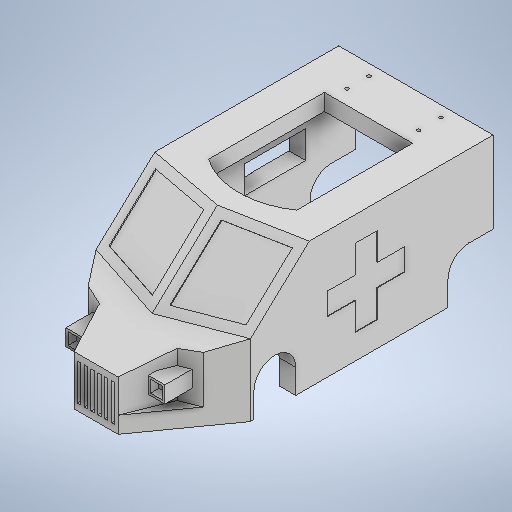
# Autodesk Inventor part: car_cover
Saved by Autodesk Inventor 2025 (Build 290162010, 162A)
## iProperties
Created: 2024-10-24
Part Number: car_cover
Material: Generic
Document SubType Name: Modeling
Designer: fist5
Density: 1 g/cm^3
Appearance: Default
Author: fist5
Autodesk Inventor part; units mm, degrees
sketch "Sketch1" plane through (0, 0, 0) normal (0, 1, 0) x (-1, 0, 0)
  line L0 (0, 0) -> (-140, 0)
  line L1 (-140, 0) -> (-140, -290)
  line L2 (-140, -290) -> (0, -290)
  line L3 (0, -290) -> (0, 0)
  line L4 (0, -70) -> (-50, 0)
  line L5 (-90, 0) -> (-140, -70)
  dimension "d0" = 290
  dimension "d1" = 140
  dimension "d2" = 70
  dimension "d3" = 50
  dimension "d4" = 50
  constraints: 12 end point, 4 point on line, 2 parallel, 1 horizontal, 1 horizontal alignment, 1 perpendicular
  measures "d0" distance between parallel lines of L2 L0
  measures "d1" distance between parallel lines of L1 L3
  measures "d2" vertical distance of L4.end L4.start
  measures "d3" distance of L0.start L4.end
  measures "d4" distance of L0.end L5.start
extrude "Extrusion1" add sketch "Sketch1" along normal blind 115 contours L4 L3 L2 L1 L5 L0
sketch "Sketch2" plane through (140, 0, -70) normal (1, 0, 0) x (0, 0, -1)
  line L0 (-70, 0) -> (-70, 115) projected
  line L1 (-70, 45) -> (0, 65)
  line L2 (0, 0) -> (0, 115) projected
  line L3 (0, 65) -> (40, 115)
  line L4 (220, 115) -> (0, 115) projected
  line L5 (-70, 0) -> (0, 0) projected
  line L6 (0, 0) -> (0, 115) projected
  line L7 (-70, 115) -> (0, 115) projected
  line L8 (-70, 0) -> (-70, 115) projected
  point P0 (0, 115)
  dimension "d7" = 20
  dimension "d8" = 45
  dimension "d9" = 40
  constraints: 4 end point, 3 point on line
  measures "d7" vertical distance of L1.start L1.end
  measures "d8" distance of L0.start L1.start
  measures "d9" horizontal distance of L3.end L1.end
extrude "Extrusion2" cut sketch "Sketch2" against normal up to next contours L0 L7 L2 L1
extrude "Extrusion3" cut sketch "Sketch2" against normal up to next contours L2 L4 L3
sketch "Sketch5" plane through (50, 45, 0) normal (0, 0.9615239, 0.2747211) x (1, 0, 0)
  line L0 (90, 72.8011) -> (-50, 72.8011) projected
  line L1 (-50, 298.0724) -> (-50, 124.9981) projected
  point P0 (-50, -12.3625)
  point P1 (20, 52.8011)
  dimension "d17" = 20
  dimension "d18" = 70
  measures "d17" distance from line of L0 point (20, 52.801)
  measures "d18" distance from line of L1 point (20, 52.801)
ref_plane "Work Plane2" through (70, 115, -110) normal (0.1294539, 0.7236066, 0.677964) x (0, -0.6837172, 0.7297471)
sketch "Sketch7" plane through (70, 115, -110) normal (0.1294539, 0.7236066, 0.677964) x (0, -0.6837172, 0.7297471)
  line L0 (0, -69.411) -> (0, 69.411) projected
  line L1 (0, 69.411) -> (-131.3545, 85.3428) projected
  line L2 (-131.3545, 85.3428) -> (-131.3545, -53.4792) projected
  line L3 (-131.3545, -53.4792) -> (0, -69.411) projected
  line L4 (63.3757, -68.2279) -> (0, -69.411) projected
  line L5 (63.3757, 70.594) -> (63.3757, -68.2279) projected
  line L6 (0, 69.411) -> (63.3757, 70.594) projected
  line L7 (0, -69.411) -> (0, 69.411) projected
  line L8 (0, 69.411) -> (63.3757, 70.594) projected
  line L9 (107.8174, 76.7345) -> (63.3757, 70.594) projected
  line L10 (107.8174, 76.7345) -> (-52.727, 96.2066) projected
  line L11 (-52.727, 96.2066) -> (-131.3545, 85.3428) projected
  line L12 (0, 69.411) -> (-131.3545, 85.3428) projected
  line L13 (128.1324, -22.955) -> (63.3757, -68.2279) projected
  line L14 (128.1324, 16.7084) -> (128.1324, -22.955) projected
  line L15 (63.3757, 70.594) -> (128.1324, 16.7084) projected
  line L16 (63.3757, 70.594) -> (63.3757, -68.2279) projected
  line L17 (63.3757, 70.594) -> (128.1324, 16.7084) projected
  line L18 (158.8997, 20.9595) -> (128.1324, 16.7084) projected
  line L19 (158.8997, 20.9595) -> (107.8174, 76.7345) projected
  line L20 (107.8174, 76.7345) -> (63.3757, 70.594) projected
  line L21 (128.1324, 16.7084) -> (128.1324, -22.955) projected
  line L22 (107.8174, -62.0875) -> (63.3757, -68.2279) projected
  line L23 (107.8174, -62.0875) -> (158.8997, -18.7039) projected
  line L24 (128.1324, 16.7084) -> (128.1324, -22.955) projected
  line L25 (158.8997, -18.7039) -> (128.1324, -22.955) projected
  line L26 (158.8997, -18.7039) -> (158.8997, 20.9595) projected
  line L27 (158.8997, 20.9595) -> (128.1324, 16.7084) projected
  line L28 (0, 0) -> (81.1658, 0)
  line L29 (81.1658, 0) -> (63.3757, 70.594)
  line L30 (0, 0) -> (63.3757, 70.594)
  point P0 (158.8997, -68.2832)
  constraints: 6 end point, 1 midpoint, 1 perpendicular
extrude "Extrusion4" cut sketch "Sketch7" along normal up to next contours L3 L2 L1 L0 | L0 L28 L5 L4 | L30 L5 L28 | L0 L6 L30 | L1 L11 L10 L9 L6
extrude "Extrusion5" add sketch "Sketch7" against normal blind 20 contours L30 L5 L28 | L5 L29 L28
ref_plane "Work Plane3" through (70, 115, -110) normal (0.1294539, -0.7236066, -0.677964) x (0, -0.6837172, 0.7297471)
sketch "Sketch9" plane through (70, 115, -110) normal (0.1294539, -0.7236066, -0.677964) x (0, -0.6837172, 0.7297471)
  line L0 (81.1658, 0) -> (63.3757, 2.3661) projected
  line L1 (-131.3545, 85.3428) -> (0, 69.411) projected
  line L2 (81.1658, 0) -> (0, 0)
  line L3 (0, 0) -> (0, 69.411)
  line L4 (0, 69.411) -> (81.1658, 69.411)
  line L5 (81.1658, 69.411) -> (81.1658, 0)
  line L6 (0, 0) -> (-9.7539, -68.2279) projected
  line L7 (0, 0) -> (-9.7539, -68.2279) projected
  line L8 (-9.7539, -68.2279) -> (-131.3545, -53.4792) projected
  line L9 (-131.3545, -53.4792) -> (-131.3545, 85.3428) projected
  line L10 (-131.3545, 85.3428) -> (0, 69.411) projected
  line L11 (0, 69.411) -> (0, 0) projected
  line L12 (0, 0) -> (81.1658, 0) projected
  line L13 (93.1192, -47.4335) -> (81.1658, 0) projected
  line L14 (148.2908, -20.1697) -> (93.1192, -47.4335) projected
  line L15 (153.1835, 20.1697) -> (148.2908, -20.1697) projected
  line L16 (63.3757, 70.594) -> (153.1835, 20.1697) projected
  line L17 (81.1658, 0) -> (63.3757, 70.594) projected
  line L18 (0, 0) -> (-9.7539, 70.594) projected
  line L19 (63.3757, 70.594) -> (0, 0) projected
  line L20 (-9.7539, 70.594) -> (63.3757, 70.594) projected
  line L21 (0, 0) -> (81.1658, 0) projected
  line L22 (0, 0) -> (-9.7539, 70.594) projected
  line L23 (63.3757, 70.594) -> (0, 0) projected
  line L24 (0, 0) -> (81.1658, 0) projected
  line L25 (0, 0) -> (-9.7539, 70.594) projected
  line L26 (63.3757, 70.594) -> (0, 0) projected
  line L27 (93.1192, -47.4335) -> (81.1658, 0) projected
  line L28 (148.2908, -20.1697) -> (93.1192, -47.4335) projected
  line L29 (153.1835, 20.1697) -> (148.2908, -20.1697) projected
  line L30 (63.3757, 70.594) -> (153.1835, 20.1697) projected
  line L31 (81.1658, 0) -> (63.3757, 70.594) projected
  line L32 (-9.7539, 70.594) -> (63.3757, 70.594) projected
  line L33 (93.1192, -47.4335) -> (81.1658, 0) projected
  line L34 (148.2908, -20.1697) -> (93.1192, -47.4335) projected
  line L35 (153.1835, 20.1697) -> (148.2908, -20.1697) projected
  line L36 (63.3757, 70.594) -> (153.1835, 20.1697) projected
  line L37 (81.1658, 0) -> (63.3757, 70.594) projected
  line L38 (-9.7539, 70.594) -> (63.3757, 70.594) projected
  point P0 (158.8997, 70.5388)
  point P1 (62.3137, 69.411)
  point P2 (63.6739, 69.411)
  point P3 (65.4828, 69.411)
  constraints: 8 end point, 2 parallel, 1 horizontal, 1 perpendicular, 1 point on line
extrude "Extrusion7" cut sketch "Sketch9" against normal blind 20 contours L20 L19 L4 L1 | L1 L3 L18 | L4 L19 L3
extrude "Extrusion8" add sketch "Sketch9" along normal blind 20 contours L19 L4 L17 L2 | L16 L4 L17 | L17 L4 L19 | L17 L4 L16 L5 | L5 L16 L15 L14 L13
sketch "Sketch10" plane through (140, 0, -290) normal (0, 0, -1) x (-1, 0, 0)
  line L0 (140, 0) -> (0, 0)
  line L1 (0, 0) -> (0, -20)
  line L2 (0, -20) -> (140, -20)
  line L3 (140, -20) -> (140, 0)
  dimension "d31" = 20
  constraints: 8 end point, 2 parallel, 1 horizontal, 1 perpendicular
  measures "d31" distance between parallel lines of L0 L2
extrude "Extrusion9" cut sketch "Sketch10" against normal up to next
ref_plane "Work Plane5" through (0, 15, 0) normal (0, -1, 0) x (1, 0, 0)
sketch "Sketch11" plane through (0, 15, 0) normal (0, -1, 0) x (1, 0, 0)
  line L0 (50, 0) -> (0, -70) projected
  line L1 (0, -70) -> (25, -63.132)
  line L2 (70, -50.7695) -> (0, -70) projected
  line L3 (25, -63.132) -> (50, 0)
  line L4 (90, 0) -> (140, -70) projected
  line L5 (90, 0) -> (140, -70)
  line L6 (140, -70) -> (70, -50.7695)
  line L7 (50, 0) -> (90, 0) projected
  line L8 (90, 0) -> (115, -63.132)
  line L9 (34.8321, -38.3031) -> (17.8321, -45.035)
  line L10 (105.1679, -38.3031) -> (122.1679, -45.035)
  line L11 (34.8321, -38.3031) -> (50, 0)
  line L12 (105.1679, -38.3031) -> (90, 0)
  line L13 (122.1679, -45.035) -> (90, 0)
  line L14 (17.8321, -45.035) -> (50, 0)
  point P0 (0, 0)
  dimension "d36" = 25
  dimension "d37" = 25
  dimension "d40" = 17
  dimension "d41" = 17
  constraints: 22 end point, 6 point on line, 4 collinear, 1 horizontal alignment, 1 perpendicular
  measures "d36" horizontal distance of L1.end L0.start
  measures "d37" horizontal distance of L8.end L4.start
  measures "d40" horizontal distance of L10.start L10.end
  measures "d41" horizontal distance of L9.start L9.end
extrude "Extrusion10" cut sketch "Sketch11" against normal up to next contours L3 L9 L0 | L4 L10 L8
ref_plane "Work Plane6" through (0, 35, 0) normal (0, -1, 0) x (1, 0, 0)
sketch "Sketch12" plane through (0, 35, 0) normal (0, -1, 0) x (1, 0, 0)
  line L0 (114.8999, -25) -> (99.8999, -25)
  line L1 (99.8999, -25) -> (99.8999, -50)
  line L2 (99.8999, -50) -> (114.8999, -50)
  line L3 (114.8999, -50) -> (114.8999, -25)
  line L4 (90, 0) -> (105.1679, -38.3031) projected
  line L5 (34.8321, -38.3031) -> (50, 0) projected
  line L6 (40.1001, -25) -> (25.1001, -25)
  line L7 (25.1001, -25) -> (25.1001, -50)
  line L8 (25.1001, -50) -> (40.1001, -50)
  line L9 (40.1001, -50) -> (40.1001, -25)
  point P0 (0, 0)
  point P1 (114.8999, -37.5)
  point P2 (99.8999, -37.5)
  point P3 (107.3999, -25)
  point P4 (107.3999, -50)
  point P5 (32.6001, -25)
  dimension "d43" = 15
  dimension "d44" = 25
  dimension "d45" = 25
  dimension "d46" = 15
  dimension "d47" = 25
  dimension "d48" = 25
  constraints: 16 end point, 5 midpoint, 4 parallel, 2 horizontal, 2 perpendicular, 2 point on line
  measures "d43" distance of point (114.9, -37.5) point (99.9, -37.5)
  measures "d44" distance of point (107.4, -25) point (107.4, -50)
  measures "d45" distance from line of L4.start L0
  measures "d46" distance between parallel lines of L7 L9
  measures "d47" vertical distance of point (0, 0) point (32.6, -25)
  measures "d48" distance between parallel lines of L6 L8
extrude "Extrusion11" add sketch "Sketch12" along normal blind 7.5 and the other way blind 7.5
sketch "Sketch13" plane through (25.1001, 27.5, -25) normal (0, 0, 1) x (1, 0, 0)
  line L0 (0, 15) -> (15, 15) projected
  line L1 (15, 15) -> (15, 0) projected
  line L2 (15, 0) -> (0, 0) projected
  line L3 (0, 0) -> (0, 15) projected
  line L4 (15, 15) -> (15, 24.6429) projected
  line L5 (15, 24.6429) -> (74.7998, 24.6429) projected
  line L6 (74.7998, 24.6429) -> (74.7998, 15) projected
  line L7 (74.7998, 0) -> (74.7998, 15) projected
  line L8 (89.7998, 0) -> (74.7998, 0) projected
  line L9 (89.7998, 15) -> (89.7998, 0) projected
  line L10 (74.7998, 15) -> (89.7998, 15) projected
  line L11 (15, -12.5) -> (15, 0) projected
  line L12 (7.0428, -12.5) -> (15, -12.5) projected
  line L13 (7.0428, -27.5) -> (7.0428, -12.5) projected
  line L14 (82.757, -27.5) -> (7.0428, -27.5) projected
  line L15 (82.757, -12.5) -> (82.757, -27.5) projected
  line L16 (74.7998, -12.5) -> (82.757, -12.5) projected
  line L17 (74.7998, 0) -> (74.7998, -12.5) projected
  line L18 (2, 15) -> (2, 0)
  line L19 (13, 15) -> (13, 0)
  line L20 (0, 13) -> (15, 13)
  line L21 (0, 2) -> (15, 2)
  line L22 (74.7998, 13) -> (89.7998, 13)
  line L23 (74.7998, 2) -> (89.7998, 2)
  line L24 (76.7998, 15) -> (76.7998, 0)
  line L25 (89.7998, 0) -> (80.0678, 0) projected
  line L26 (87.7998, 15) -> (87.7998, 0)
  line L27 (2, 13) -> (13, 13)
  line L28 (13, 13) -> (13, 2)
  line L29 (13, 2) -> (2, 2)
  line L30 (2, 2) -> (2, 13)
  line L31 (76.7998, 13) -> (87.7998, 13)
  line L32 (87.7998, 13) -> (87.7998, 2)
  line L33 (87.7998, 2) -> (76.7998, 2)
  line L34 (76.7998, 2) -> (76.7998, 13)
  line L35 (0, 15) -> (15, 15) projected
  line L36 (0, 15) -> (15, 15)
  line L37 (15, 15) -> (15, 0)
  line L38 (15, 0) -> (0, 0)
  line L39 (0, 0) -> (0, 15)
  line L40 (74.7998, 15) -> (80.0678, 15) projected
  line L41 (74.7998, 15) -> (89.7998, 15)
  line L42 (89.7998, 15) -> (89.7998, 0)
  line L43 (89.7998, 0) -> (74.7998, 0)
  line L44 (74.7998, 0) -> (74.7998, 15)
  point P0 (-25.1001, -27.5)
  point P1 (7.5, 0)
  point P2 (7.5, 2)
  point P3 (87.7998, 13)
  point P4 (13, 13)
  point P5 (2, 2)
  dimension "d53" = 2
  dimension "d54" = 11
  dimension "d55" = 2
  dimension "d56" = 11
  dimension "d57" = 2
  dimension "d58" = 11
  dimension "d59" = 2
  dimension "d60" = 2
  constraints: 48 end point, 24 point on line, 10 perpendicular, 8 parallel, 5 horizontal, 2 midpoint, 1 vertical
  measures "d53" distance of point (7.5, 0) point (7.5, 2)
  measures "d54" distance between parallel lines of L21 L20
  measures "d55" distance between parallel lines of L3 L18
  measures "d56" distance between parallel lines of L18 L19
  measures "d57" distance between parallel lines of L9 L26
  measures "d58" distance between parallel lines of L26 L24
  measures "d59" distance between parallel lines of L10 L22
  measures "d60" distance between parallel lines of L8 L23
extrude "Extrusion12" add sketch "Sketch13" along normal blind 7.5 contours L0 L18 L20 L3 | L0 L19 L20 L18 | L20 L18 L21 L3 | L0 L1 L20 L19 | L21 L18 L2 L3 | L20 L1 L21 L19 | L21 L19 L2 L18 | L21 L1 L2 L19 | L10 L24 L22 L7 | L22 L24 L23 L7 | L10 L26 L22 L24 | L23 L24 L8 L7 | L23 L26 L8 L24 | L26 L10 L9 L22 | L22 L9 L23 L26 | L23 L9 L8 L26
sketch "Sketch14" plane through (50, 0, 0) normal (0, 0, 1) x (1, 0, 0)
  line L0 (3.0769, 39) -> (6.1538, 39)
  line L1 (6.1538, 39) -> (6.1538, 6)
  line L2 (6.1538, 6) -> (3.0769, 6)
  line L3 (3.0769, 6) -> (3.0769, 39)
  line L4 (9.2308, 39) -> (12.3077, 39)
  line L5 (12.3077, 39) -> (12.3077, 6)
  line L6 (12.3077, 6) -> (9.2308, 6)
  line L7 (9.2308, 6) -> (9.2308, 39)
  line L8 (15.3846, 39) -> (18.4615, 39)
  line L9 (18.4615, 39) -> (18.4615, 6)
  line L10 (18.4615, 6) -> (15.3846, 6)
  line L11 (15.3846, 6) -> (15.3846, 39)
  line L12 (21.5385, 39) -> (24.6154, 39)
  line L13 (24.6154, 39) -> (24.6154, 6)
  line L14 (24.6154, 6) -> (21.5385, 6)
  line L15 (21.5385, 6) -> (21.5385, 39)
  line L16 (27.6923, 39) -> (30.7692, 39)
  line L17 (30.7692, 39) -> (30.7692, 6)
  line L18 (30.7692, 6) -> (27.6923, 6)
  line L19 (27.6923, 6) -> (27.6923, 39)
  line L20 (33.8462, 39) -> (36.9231, 39)
  line L21 (36.9231, 39) -> (36.9231, 6)
  line L22 (36.9231, 6) -> (33.8462, 6)
  line L23 (33.8462, 6) -> (33.8462, 39)
  line L24 (0, 15) -> (0, 45) projected
  line L25 (40, 45) -> (0, 45) projected
  line L26 (0, 0) -> (40, 0) projected
  point P0 (-50, 0)
  point P1 (16.9231, 39)
  point P2 (35.3846, 6)
  dimension "d63" = 3.0769
  dimension "d64" = 3.0769
  dimension "d65" = 3.0769
  dimension "d66" = 3.0769
  dimension "d67" = 3.0769
  dimension "d68" = 3.0769
  dimension "d69" = 3.0769
  dimension "d70" = 3.0769
  dimension "d71" = 3.0769
  dimension "d72" = 3.0769
  dimension "d73" = 3.0769
  dimension "d74" = 3.0769
  dimension "d75" = 6
  dimension "d76" = 6
  constraints: 48 end point, 12 parallel, 9 point on line, 6 horizontal, 6 perpendicular, 2 midpoint, 1 horizontal alignment
  measures "d63" distance between parallel lines of L24 L3
  measures "d64" distance between parallel lines of L7 L1
  measures "d65" distance between parallel lines of L11 L5
  measures "d66" distance between parallel lines of L3 L1
  measures "d67" distance between parallel lines of L11 L9
  measures "d68" distance between parallel lines of L9 L15
  measures "d69" distance between parallel lines of L7 L5
  measures "d70" distance between parallel lines of L13 L15
  measures "d71" distance between parallel lines of L13 L19
  measures "d72" distance between parallel lines of L19 L17
  measures "d73" distance between parallel lines of L17 L23
  measures "d74" distance between parallel lines of L23 L21
  measures "d75" distance from line of point (16.923, 39) L25
  measures "d76" distance from line of L26 point (35.385, 6)
extrude "Extrusion13" cut sketch "Sketch14" against normal blind 7.5
sketch "Sketch15" plane through (70, 115, -110) normal (0.1294539, 0.7236066, 0.677964) x (0.9915854, -0.0944686, -0.0885098)
  line L0 (8, -6.9706) -> (62.594, 0.5726)
  line L1 (62.594, 0.5726) -> (62.594, -57.1417)
  line L2 (62.594, -57.1417) -> (8, -70.8996)
  line L3 (8, -70.8996) -> (8, -6.9706)
  line L4 (0, 0) -> (0, -81.1658) projected
  line L5 (0, 0) -> (70.594, 9.7539) projected
  line L6 (70.594, 9.7539) -> (70.594, -63.3757) projected
  line L7 (70.594, -63.3757) -> (0, -81.1658) projected
  point P0 (-68.2832, -158.8997)
  dimension "d79" = 8
  dimension "d80" = 8
  dimension "d81" = 8
  dimension "d82" = 8
  constraints: 8 end point, 4 parallel
  measures "d79" distance between parallel lines of L5 L0
  measures "d80" distance between parallel lines of L6 L1
  measures "d81" distance between parallel lines of L7 L2
  measures "d82" distance between parallel lines of L4 L3
extrude "Extrusion14" cut sketch "Sketch15" against normal blind 1 contours L0 L1 L2 L3
sketch "Sketch16" plane through (70, 115, -110) normal (-0.1294539, 0.7236066, 0.677964) x (0.9915854, 0.0944686, 0.0885098)
  line L0 (-8, -70.8996) -> (-62.594, -57.1417)
  line L1 (-62.594, -57.1417) -> (-62.594, 0.5726)
  line L2 (-62.594, 0.5726) -> (-8, -6.9706)
  line L3 (-8, -6.9706) -> (-8, -70.8996)
  line L4 (-70.594, 9.7539) -> (0, 0) projected
  line L5 (0, 0) -> (0, -81.1658) projected
  line L6 (0, -81.1658) -> (-70.594, -63.3757) projected
  line L7 (-70.594, -63.3757) -> (-70.594, 9.7539) projected
  point P0 (-70.5388, -158.8997)
  point P1 (0, -40.5829)
  dimension "d85" = 8
  dimension "d86" = 8
  dimension "d87" = 8
  dimension "d88" = 8
  constraints: 8 end point, 5 parallel, 1 midpoint, 1 vertical
  measures "d85" distance between parallel lines of L4 L2
  measures "d86" distance between parallel lines of L7 L1
  measures "d87" distance between parallel lines of L6 L0
  measures "d88" distance from line of point (0, -40.583) L3
extrude "Extrusion15" cut sketch "Sketch16" against normal blind 1 contours L0 L1 L2 L3
sketch "Sketch17" plane through (0, 0, 0) normal (0, -1, 0) x (1, 0, 0)
  line L0 (90, 0) -> (140, -70) projected
  line L1 (140, -70) -> (140, -290) projected
  line L2 (140, -290) -> (0, -290) projected
  line L3 (0, -290) -> (0, -70) projected
  line L4 (0, -70) -> (50, 0) projected
  line L5 (50, 0) -> (90, 0) projected
  line L6 (0, -123.3662) -> (70, -110) projected
  line L7 (70, -110) -> (140, -123.3662) projected
  line L8 (140, -123.3662) -> (140, -290) projected
  line L9 (140, -290) -> (0, -290) projected
  line L10 (0, -290) -> (0, -123.3662) projected
  line L11 (125, -290) -> (15, -290)
  line L12 (15, -290) -> (15, -120.502)
  line L13 (15, -120.502) -> (125, -120.502)
  line L14 (125, -120.502) -> (125, -290)
  line L15 (140, -70) -> (0, -70)
  line L16 (131.9379, -116.636) -> (131.9379, -74.5192) projected
  line L17 (140, -290) -> (0, -290) projected
  point P0 (0, 0)
  point P1 (125, -205.251)
  point P2 (15, -290)
  dimension "d91" = 15
  dimension "d92" = 15
  constraints: 10 end point, 2 parallel, 2 perpendicular, 2 point on line, 1 horizontal, 1 midpoint
  measures "d91" distance from line of point (125, -205.251) L1
  measures "d92" distance between parallel lines of L3 L12
extrude "Extrusion16" cut sketch "Sketch17" against normal blind 100 contours L14 L2 L12 L13
sketch "Sketch18" plane through (0, 0, 0) normal (0, -1, 0) x (1, 0, 0)
  line L0 (0, -123.3662) -> (70, -110) projected
  line L1 (15, -120.502) -> (15, -72.6132)
  line L2 (62.1968, -59.6473) -> (8.0621, -74.5192) projected
  line L3 (70, -110) -> (140, -123.3662) projected
  line L4 (125, -120.502) -> (125, -71.8997)
  line L5 (132.0673, -73.8412) -> (77.9327, -58.9693) projected
  line L6 (125, -120.502) -> (125, -290) projected
  line L7 (15, -290) -> (15, -120.502) projected
  line L8 (70, -110) -> (70, -50.7695) projected
  line L9 (125, -71.8997) -> (70, -50.7695)
  line L10 (70, -50.7695) -> (15, -72.6132)
  line L11 (125, -120.502) -> (15, -120.502)
  point P0 (0, 0)
  constraints: 10 end point, 6 point on line, 1 parallel, 1 perpendicular, 1 vertical
extrude "Extrusion17" cut sketch "Sketch18" against normal blind 55
chamfer "Chamfer1" distance 45 angle 45 1 edges at (70, 55, -120.502)
sketch "Sketch19" plane through (0, 115, 0) normal (0, 1, 0) x (1, 0, 0)
  line L0 (110, 247) -> (30, 247)
  line L1 (30, 247) -> (30, 142)
  line L2 (30, 142) -> (110, 142)
  line L3 (110, 142) -> (110, 247)
  line L4 (140, 290) -> (0, 290) projected
  line L5 (0, 290) -> (0, 123.3662) projected
  line L6 (140, 123.3662) -> (140, 290) projected
  point P0 (0, 0)
  point P1 (0, 206.6831)
  dimension "d100" = 43
  dimension "d101" = 30
  dimension "d102" = 30
  dimension "d103" = 105
  constraints: 8 end point, 2 parallel, 1 horizontal, 1 midpoint, 1 perpendicular
  measures "d100" distance between parallel lines of L4 L0
  measures "d101" distance from line of point (0, 206.683) L1
  measures "d102" distance between parallel lines of L6 L3
  measures "d103" distance between parallel lines of L0 L2
extrude "Extrusion18" cut sketch "Sketch19" against normal up to next
sketch "Sketch20" plane through (0, 0, -290) normal (-1, 0, 0) x (0, 0, 1)
  circle A0 centre (22, 22.1) radius 19
  circle A1 centre (198, 22.1) radius 19
  line L0 (0, 0) -> (220, 0) projected
  line L1 (0, 0) -> (0, 115) projected
  line L2 (0, 0) -> (0, 115) projected
  line L3 (22, 41.1) -> (0, 41.1)
  line L4 (41, 22.1) -> (41, 0)
  line L5 (218.1003, 0) -> (0, 0) projected
  line L6 (179, 22.1) -> (179, 0)
  line L7 (217.3868, 0) -> (217.3868, 55) projected
  line L8 (217, 22.1) -> (217, 0)
  point P0 (290, 0)
  dimension "d106" = 22.1
  dimension "d107" = 22.1
  dimension "d108" = 22
  dimension "d109" = 198
  dimension "d110" = 38
  dimension "d111" = 38
  constraints: 8 end point, 4 perpendicular, 4 point on circle, 4 point on line, 3 tangent, 2 centre point, 1 horizontal alignment
  measures "d106" distance from line of L0 A1.centre
  measures "d107" distance from line of L0 A0.centre
  measures "d108" distance from line of L1 A0.centre
  measures "d109" distance from line of L1 A1.centre
  measures "d110" diameter of A0
  measures "d111" diameter of A1
extrude "Extrusion19" cut sketch "Sketch20" against normal up to surface (140 mm away)
sketch "Sketch21" plane through (0, 0, -70) normal (-1, 0, 0) x (0, 0, 1)
  line L0 (-140, 67.5) -> (-70, 67.5)
  line L1 (-70, 67.5) -> (-70, 47.5)
  line L2 (-70, 47.5) -> (-140, 47.5)
  line L3 (-140, 47.5) -> (-140, 67.5)
  line L4 (-115, 92.5) -> (-95, 92.5)
  line L5 (-95, 92.5) -> (-95, 22.5)
  line L6 (-95, 22.5) -> (-115, 22.5)
  line L7 (-115, 22.5) -> (-115, 92.5)
  line L8 (-179, 0) -> (-41, 0) projected
  line L9 (-220, 41.1) -> (-220, 115) projected
  point P0 (70, 0)
  point P1 (-95, 57.5)
  point P2 (-105, 67.5)
  point P3 (-140, 57.5)
  point P4 (-70, 57.5)
  point P5 (-105, 92.5)
  point P6 (-115, 67.5)
  point P7 (-115, 47.5)
  point P8 (-95, 47.5)
  point P9 (-95, 67.5)
  dimension "d114" = 57.5
  dimension "d115" = 115
  dimension "d116" = 70
  dimension "d117" = 70
  dimension "d118" = 20
  dimension "d119" = 20
  constraints: 16 end point, 5 midpoint, 4 parallel, 2 horizontal, 2 perpendicular, 1 horizontal alignment, 1 vertical alignment
  measures "d114" distance from line of L8 point (-95, 57.5)
  measures "d115" distance from line of L9 point (-105, 67.5)
  measures "d116" distance between parallel lines of L6 L4
  measures "d117" distance of point (-140, 57.5) point (-70, 57.5)
  measures "d118" distance between parallel lines of L2 L0
  measures "d119" distance between parallel lines of L7 L5
extrude "Extrusion20" cut sketch "Sketch21" against normal blind 0.5
sketch "Sketch22" plane through (140, 0, -70) normal (1, 0, 0) x (0, 0, -1)
  line L0 (115, 67.5) -> (115, 92.5) projected
  line L1 (140, 67.5) -> (115, 67.5) projected
  line L2 (140, 47.5) -> (140, 67.5) projected
  line L3 (115, 47.5) -> (140, 47.5) projected
  line L4 (115, 22.5) -> (115, 47.5) projected
  line L5 (95, 22.5) -> (115, 22.5) projected
  line L6 (95, 47.5) -> (95, 22.5) projected
  line L7 (70, 47.5) -> (95, 47.5) projected
  line L8 (70, 67.5) -> (70, 47.5) projected
  line L9 (95, 67.5) -> (70, 67.5) projected
  line L10 (95, 92.5) -> (95, 67.5) projected
  line L11 (115, 92.5) -> (95, 92.5) projected
  point P0 (-70, 0)
extrude "Extrusion21" cut sketch "Sketch22" against normal blind 0.5
sketch "Sketch23" plane through (0, 115, 0) normal (0, 1, 0) x (1, 0, 0)
  line L0 (102.5, 280) -> (37.5, 280)
  line L1 (37.5, 280) -> (37.5, 260)
  line L2 (37.5, 260) -> (102.5, 260)
  line L3 (102.5, 260) -> (102.5, 280)
  line L4 (0, 290) -> (0, 123.3662) projected
  line L5 (140, 290) -> (0, 290) projected
  circle A0 centre (102.5, 260) radius 1.5
  point P0 (0, 0)
  point P1 (70, 280)
  point P2 (37.5, 270)
  point P3 (102.5, 270)
  dimension "d124" = 70
  dimension "d125" = 65
  dimension "d126" = 20
  dimension "d127" = 20
  dimension "d128" = 3
  constraints: 8 end point, 3 midpoint, 2 parallel, 1 centre point, 1 coincident, 1 horizontal, 1 perpendicular
  measures "d124" distance from line of L4 point (70, 280)
  measures "d125" distance of point (37.5, 270) point (102.5, 270)
  measures "d126" distance between parallel lines of L0 L2
  measures "d127" distance from line of L5 point (37.5, 270)
  measures "d128" diameter of A0
extrude "Extrusion22" cut sketch "Sketch23" against normal up to next contours A0 L2 L3 | L3 L2 A0
pattern_linear "Rectangular Pattern1" count 2 spacing 65 along (-1, 0, 0) count 2 spacing 20 along (0, 0, -1) of "Extrusion22"
sketch "Sketch24" plane through (0, 0, 0) normal (0, -1, 0) x (1, 0, 0)
  line L0 (132.5, -235) -> (132.5, -134.3405)
  line L1 (7.5, -235) -> (7.5, -134.3405)
  line L2 (140, -290) -> (125, -290) projected
  line L3 (15, -290) -> (0, -290) projected
  line L4 (125, -111) -> (125, -249) projected
  line L5 (0, -249) -> (0, -111) projected
  circle A0 centre (132.5, -235) radius 1.5
  circle A1 centre (7.5, -235) radius 1.5
  point P0 (0, 0)
  point P1 (132.5, -290)
  dimension "d137" = 55
  dimension "d138" = 55
  dimension "d139" = 7.5
  dimension "d140" = 7.5
  dimension "d141" = 3
  dimension "d142" = 3
  constraints: 4 end point, 2 centre point, 2 coincident, 2 vertical, 1 midpoint
  measures "d137" distance of point (132.5, -290) L0.start
  measures "d138" distance from line of L3 L1.start
  measures "d139" distance between parallel lines of L4 L0
  measures "d140" distance between parallel lines of L1 L5
  measures "d141" diameter of A1
  measures "d142" diameter of A0
extrude "Extrusion23" cut sketch "Sketch24" against normal blind 15
pattern_linear "Rectangular Pattern2" count 8 spacing 15 along (0, 0, 1) of "Extrusion23"
sketch "Sketch25" plane through (0, 0, -70) normal (-1, 0, 0) x (0, 0, 1)
  line L0 (-175, 80) -> (-120, 80)
  line L1 (-120, 80) -> (-120, 55)
  line L2 (-120, 55) -> (-175, 55)
  line L3 (-175, 55) -> (-175, 80)
  line L4 (-179, 0) -> (-41, 0) projected
  line L5 (-220, 41.1) -> (-220, 115) projected
  point P0 (70, 0)
  point P1 (-120, 67.5)
  dimension "d148" = 80
  dimension "d149" = 55
  dimension "d150" = 45
  dimension "d151" = 100
  constraints: 8 end point, 2 parallel, 1 horizontal, 1 midpoint, 1 perpendicular
  measures "d148" distance between parallel lines of L4 L0
  measures "d149" distance between parallel lines of L4 L2
  measures "d150" distance between parallel lines of L5 L3
  measures "d151" distance from line of L5 point (-120, 67.5)
extrude "Extrusion24" cut sketch "Sketch25" against normal up to surface (15 mm away)
sketch "Sketch26" plane through (0, 115, 0) normal (0, 1, 0) x (1, 0, 0)
  circle A0 centre (70, 199.5776) radius 70.1084
  line L0 (110, 142) -> (110, 247) projected
  line L1 (110, 142) -> (30, 142)
  circle A1 centre (102.5, 260) radius 1.5 projected
  point P0 (0, 0)
  constraints: 2 end point, 2 point on circle, 1 centre point, 1 perpendicular, 1 tangent
extrude "Extrusion25" cut sketch "Sketch26" against normal up to surface (15 mm away) contours L1 A0 picked at (80.2779, 140.2045)
body "Solid1"
